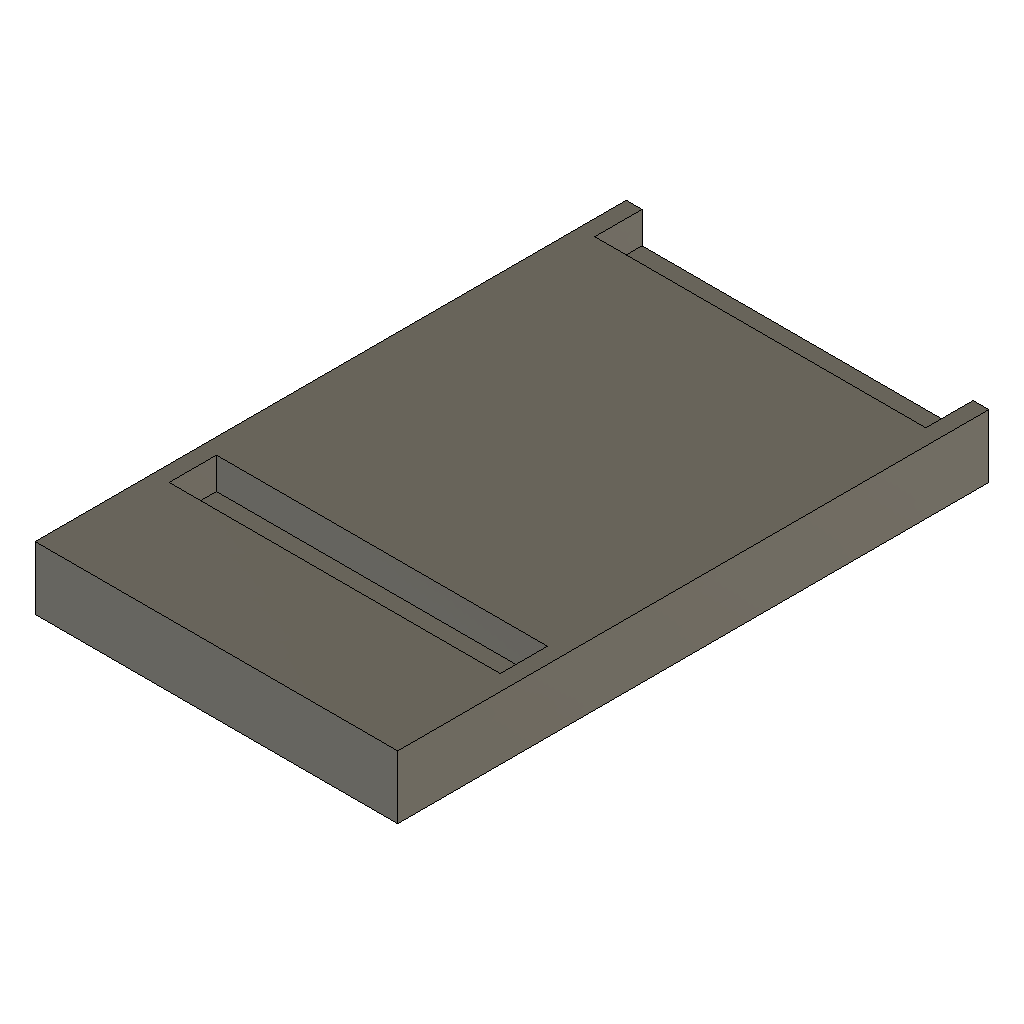
Charger Mount (Autodesk Fusion 360 design; units mm, degrees)
Autodesk Fusion 360 part; units mm, degrees
sketch "Sketch1" plane through (0, 0, 0) normal (0, 0, 1) x (1, 0, 0)
  line L0 (0, 0) -> (23, 0)
  line L1 (23, 0) -> (23, 37.5)
  line L2 (23, 37.5) -> (0, 37.5)
  line L3 (0, 37.5) -> (0, 0)
  dimension "d1" = 23
  dimension "d2" = 37.5
  constraint horizontal L0
  constraint vertical L1
  constraint horizontal L2
  constraint vertical L3
  constraint coincident L0.start L3.end
  measures "d1" distance of L0.start L0.end
  measures "d2" distance of L0.start L2.end
extrude "Extrude1" add sketch "Sketch1" along normal blind 4
sketch "Sketch2" plane through (0, 0, 4) normal (0, 0, 1) x (-1, 0, 0)
  line L0 (0, -37.5) -> (0, 0)
  line L1 (0, 0) -> (-23, 0)
  line L2 (-23, 0) -> (-23, -37.5)
  line L3 (-23, -37.5) -> (0, -37.5)
  line L4 (-1, -7.5) -> (-22, -7.5)
  line L5 (-22, -7.5) -> (-22, -10.5)
  line L6 (-22, -10.5) -> (-1, -10.5)
  line L7 (-1, -10.5) -> (-1, -7.5)
  line L8 (-1, -37.5) -> (-22, -37.5)
  line L9 (-22, -37.5) -> (-22, -34.5)
  line L10 (-22, -34.5) -> (-1, -34.5)
  line L11 (-1, -34.5) -> (-1, -37.5)
  dimension "d5" = 21
  dimension "d6" = 3
  dimension "d7" = 1
  dimension "d37" = 21
  dimension "d38" = 3
  dimension "d40" = 1
  dimension "d41" = 24
  dimension "d42" = 7.5
  constraint horizontal L4
  constraint vertical L5
  constraint horizontal L6
  constraint vertical L7
  constraint horizontal L8
  constraint vertical L9
  constraint horizontal L10
  constraint vertical L11
  measures "d5" distance of L4.start L4.end
  measures "d6" distance of L4.start L6.end
  measures "d7" distance of L2 L5
  measures "d37" distance of L8.start L8.end
  measures "d38" distance of L8.start L10.end
  measures "d40" distance of L0 L11
  measures "d41" distance of L6 L10
  measures "d42" distance of L1 L4
extrude "Extrude2" cut sketch "Sketch2" against normal blind 2 contours L3 L8 L9 L10 L11 | L4 L5 L6 L7
